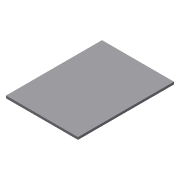
# Autodesk Inventor part: 00_Metalsheet_1mm_30x40
Saved by Autodesk Inventor 2019 (Build 230136000, 136)
## iProperties
Created: 2019-06-11
Part Number: 00_Metalsheet_1mm_30x40
Material: Generic
Document SubType Name: Modeling
Designer: diederichbenedict
Density: 1 g/cm^3
Appearance: Default
Author: diederichbenedict
Autodesk Inventor part; units mm, degrees
ref_plane "YZ Plane" through (0, 0, 0) normal (1, 0, 0) x (0, 1, 0)
ref_plane "XZ Plane" through (0, 0, 0) normal (0, 1, 0) x (-1, 0, 0)
ref_plane "XY Plane" through (0, 0, 0) normal (0, 0, 1) x (1, 0, 0)
sketch "Sketch1" plane through (0, 0, 0) normal (0, 1, 0) x (-1, 0, 0)
  line L0 (3.043, 57.9959) -> (-26.957, 57.9959)
  line L1 (-26.957, 57.9959) -> (-26.957, 17.9959)
  line L2 (-26.957, 17.9959) -> (3.043, 17.9959)
  line L3 (3.043, 17.9959) -> (3.043, 57.9959)
  point P0 (0, 0)
  dimension "d0" = 30
  dimension "d1" = 40
  constraints: 8 end point, 2 parallel, 1 horizontal, 1 perpendicular
  measures "d0" distance of L2.end L1.end
  measures "d1" distance of L1.end L0.end
extrude "Extrusion1" add sketch "Sketch1" along normal blind 1
body "Solid1"
